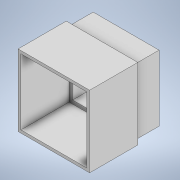
# Autodesk Inventor part: IMX178 Camera Case Cap
Saved by Autodesk Inventor 2022.1 (Build 261234000, 234)
## iProperties
Created: 2021-07-23
Part Number: IMX178 Camera Case Cap
Material: Generic
Document SubType Name: Modeling
Designer: robst
Density: 1 g/cm^3
Appearance: Default
Author: robst
Autodesk Inventor part; units mm, degrees
ref_plane "YZ Plane" through (0, 0, 0) normal (1, 0, 0) x (0, 1, 0)
ref_plane "XZ Plane" through (0, 0, 0) normal (0, 1, 0) x (-1, 0, 0)
ref_plane "XY Plane" through (0, 0, 0) normal (0, 0, 1) x (1, 0, 0)
sketch "Sketch18" plane through (0, 0, 0) normal (0, 0, 1) x (1, 0, 0)
  line L0 (-23.25, -23.25) -> (23.25, -23.25)
  line L1 (23.25, -23.25) -> (23.25, 23.25)
  line L2 (23.25, 23.25) -> (-23.25, 23.25)
  line L3 (-23.25, 23.25) -> (-23.25, -23.25)
  line L4 (-23.25, -23.25) -> (23.25, 23.25) construction
  line L5 (23.25, -23.25) -> (-23.25, 23.25) construction
  line L6 (-20.75, -20.75) -> (20.75, -20.75)
  line L7 (20.75, -20.75) -> (20.75, 20.75)
  line L8 (20.75, 20.75) -> (-20.75, 20.75)
  line L9 (-20.75, 20.75) -> (-20.75, -20.75)
  line L10 (-20.75, -20.75) -> (20.75, 20.75) construction
  line L11 (20.75, -20.75) -> (-20.75, 20.75) construction
  circle A0 centre (0, 0) radius 2.6
  dimension "d102" = 46.5
  dimension "d103" = 46.5
  dimension "d104" = 2.5
  dimension "d105" = 2.5
  dimension "d106" = 5.2
  constraints: 24 end point, 4 midpoint, 4 parallel, 2 horizontal, 2 perpendicular, 1 centre point, 1 coincident
  measures "d102" distance of L1.end L2.end
  measures "d103" distance of L2.end L0.start
  measures "d104" distance between parallel lines of L8 L2
  measures "d105" distance between parallel lines of L9 L3
  measures "d106" diameter of A0
extrude "Extrusion14" add sketch "Sketch18" against normal blind 2 contours L3 L2 L1 L0 | L9 L8 L7 L6 | A0
extrude "Extrusion15" add sketch "Sketch18" along normal blind 15 contours L3 L2 L1 L0
sketch "Sketch19" plane through (0, 0, 15) normal (0, 0, 1) x (1, 0, 0)
  line L0 (-20.75, -20.75) -> (20.75, -20.75)
  line L1 (20.75, -20.75) -> (20.75, 20.75)
  line L2 (20.75, 20.75) -> (-20.75, 20.75)
  line L3 (-20.75, 20.75) -> (-20.75, -20.75)
  line L4 (-20.75, -20.75) -> (20.75, 20.75) construction
  line L5 (20.75, -20.75) -> (-20.75, 20.75) construction
  line L6 (-25.25, -25.25) -> (25.25, -25.25)
  line L7 (25.25, -25.25) -> (25.25, 25.25)
  line L8 (25.25, 25.25) -> (-25.25, 25.25)
  line L9 (-25.25, 25.25) -> (-25.25, -25.25)
  line L10 (-25.25, -25.25) -> (25.25, 25.25) construction
  line L11 (25.25, -25.25) -> (-25.25, 25.25) construction
  line L12 (23.25, -23.25) -> (23.25, 23.25) projected
  line L13 (23.25, 23.25) -> (-23.25, 23.25) projected
  line L14 (-23.25, 23.25) -> (-23.25, -23.25) projected
  line L15 (-23.25, -23.25) -> (23.25, -23.25) projected
  point P0 (0, 0)
  dimension "d111" = 2
  dimension "d112" = 2
  constraints: 24 end point, 4 midpoint, 4 parallel, 2 perpendicular, 1 horizontal
  measures "d111" distance between parallel lines of L7 L12
  measures "d112" distance between parallel lines of L8 L13
extrude "Extrusion16" add sketch "Sketch19" along normal blind 34 contours L9 L8 L7 L6
equation "\"screwSpacing\" = 34"
equation "\"interiorWidth\" = 42"
equation "\"wallThickness\" = 2"
equation "\"holeDiameter\" = 3"
body "Solid7"
